Autodesk Fusion 360 part; units mm, degrees
(part 2 of 3)
  point P42 (0.5082, -2.6613)
  point P43 (0.8246, -2.9842)
  point P44 (1.3977, -3.4768)
  point P45 (1.9615, -3.8935)
  point P46 (4.9792, -5.5211)
  point P47 (9.2288, -7.083)
  point P48 (14.7308, -8.5341)
  point P49 (21.5325, -9.8694)
  point P50 (29.688, -11.1157)
  point P51 (39.2683, -12.4107)
  point P52 (50.1896, -13.9731)
  point P53 (62.2459, -15.9385)
  point P54 (75.2086, -18.3956)
  point P55 (88.7376, -21.406)
  point P56 (102.4623, -24.7749)
  point P57 (116.1281, -28.2634)
  point P58 (129.5519, -31.7626)
  point P59 (142.5417, -35.2316)
  point P60 (154.8635, -38.6462)
  point P61 (166.2937, -41.9413)
  point P62 (176.6711, -45.0342)
  point P63 (185.8834, -47.8702)
  point P64 (193.8319, -50.4036)
  point P65 (200.448, -52.5873)
  point P66 (205.676, -54.3931)
  point P67 (209.4523, -55.7878)
  point P68 (211.7241, -56.7102)
  point P69 (293.9, -147.2)
  point P70 (294.0652, -146.0004)
  point P71 (294.1279, -145.0895)
  point P72 (294.0772, -144.1146)
  point P73 (293.9994, -143.1676)
  point P74 (293.9127, -142.2878)
  point P75 (293.7566, -141.3589)
  point P76 (293.5926, -140.4177)
  point P77 (293.4026, -139.4808)
  point P78 (293.2255, -138.6248)
  point P79 (293.0974, -137.8749)
  point P80 (292.9375, -137.1059)
  point P81 (292.7021, -136.2377)
  point P82 (292.4834, -135.3764)
  point P83 (292.2718, -134.5094)
  point P84 (292.0197, -133.588)
  point P85 (291.7467, -132.6417)
  point P86 (291.4876, -131.7273)
  point P87 (291.2208, -130.8227)
  point P88 (290.9286, -129.8942)
  point P89 (290.6361, -128.9678)
  point P90 (290.3438, -128.0412)
  point P91 (290.0291, -127.0895)
  point P92 (289.6941, -126.1123)
  point P93 (289.3385, -125.1082)
  point P94 (288.9614, -124.0797)
  point P95 (288.5631, -123.025)
  point P96 (288.1588, -121.9764)
  point P97 (287.7553, -120.927)
  point P98 (287.3046, -119.8315)
  point P99 (286.8381, -118.7059)
  point P100 (286.3461, -117.5584)
  point P101 (285.8275, -116.3901)
  point P102 (285.287, -115.1981)
  point P103 (284.7, -113.9592)
  point P104 (284.1126, -112.7207)
  point P105 (283.4966, -111.4635)
  point P106 (282.8531, -110.1882)
  point P107 (282.2008, -108.9218)
  point P108 (281.514, -107.6427)
  point P109 (280.8144, -106.3767)
  point P110 (280.1033, -105.1225)
  point P111 (279.3817, -103.8791)
  point P112 (278.6514, -102.6445)
  point P113 (277.9115, -101.4197)
  point P114 (277.1545, -100.2124)
  point P115 (276.3791, -99.0239)
  point P116 (275.5907, -97.8488)
  point P117 (274.7985, -96.6775)
  point P118 (273.9974, -95.5153)
  point P119 (273.1825, -94.3673)
  point P120 (272.3507, -93.2365)
  point P121 (271.5048, -92.1202)
  point P122 (270.6449, -91.018)
  point P123 (269.7704, -89.9293)
  point P124 (268.8852, -88.853)
  point P125 (267.9907, -87.7864)
  point P126 (267.0817, -86.7346)
  point P127 (266.1565, -85.6976)
  point P128 (265.2171, -84.6768)
  point P129 (264.2633, -83.6708)
  point P130 (263.2951, -82.6778)
  point P131 (262.3106, -81.7032)
  point P132 (261.3066, -80.7468)
  point P133 (260.2862, -79.8089)
  point P134 (259.248, -78.8874)
  point P135 (258.1963, -77.9799)
  point P136 (257.1267, -77.0922)
  point P137 (256.0425, -76.2178)
  point P138 (254.9438, -75.3584)
  point P139 (253.8335, -74.5123)
  point P140 (252.7072, -73.681)
  point P141 (251.5643, -72.8667)
  point P142 (250.4037, -72.0704)
  point P143 (249.2245, -71.2932)
  point P144 (248.0274, -70.5343)
  point P145 (246.812, -69.7941)
  point P146 (245.5815, -69.0694)
  point P147 (244.3299, -68.3662)
  point P148 (243.0593, -67.6824)
  point P149 (241.7646, -67.0233)
  point P150 (240.4487, -66.3841)
  point P151 (239.1158, -65.7641)
  point P152 (237.8237, -65.1966)
  point P153 (236.6088, -64.6907)
  point P154 (235.4954, -64.2713)
  point P155 (234.4319, -63.8934)
  point P156 (233.39, -63.5413)
  point P157 (232.3995, -63.231)
  point P158 (231.4612, -62.9634)
  point P159 (230.5496, -62.7129)
  point P160 (229.667, -62.4825)
  point P161 (228.8288, -62.2994)
  point P162 (227.9917, -62.1167)
  point P163 (227.1763, -61.9564)
  point P164 (226.3862, -61.82)
  point P165 (225.5929, -61.6851)
  point P166 (224.818, -61.5795)
  point P167 (224.0639, -61.5005)
  point P168 (223.3078, -61.4218)
  point P169 (222.5837, -61.3585)
  point P170 (221.9248, -61.3226)
  point P171 (221.2934, -61.3067)
  point P172 (220.635, -61.2704)
  point P173 (220.0004, -61.2578)
  point P174 (219.4199, -61.2841)
  point P175 (218.8468, -61.3011)
  point P176 (218.2642, -61.3296)
  point P177 (217.6776, -61.3621)
  point P178 (217.0805, -61.4037)
  point P179 (216.5149, -61.4628)
  point P180 (215.9731, -61.542)
  point P181 (215.4331, -61.6212)
  point P182 (214.8778, -61.716)
  point P183 (214.3167, -61.8167)
  point P184 (213.7818, -61.937)
  point P185 (213.2797, -62.0717)
  point P186 (212.7808, -62.2013)
  point P187 (212.2834, -62.3312)
  point P188 (211.821, -62.4733)
  point P189 (211.3771, -62.6427)
  point P190 (210.9196, -62.8243)
  point P191 (210.4453, -63.0248)
  point P192 (209.9732, -63.2711)
  point P193 (209.4657, -63.5038)
  point P194 (208.9678, -63.7748)
  point P195 (208.5001, -64.0628)
  point P196 (208.135, -64.3865)
  point P197 (207.804, -64.725)
  point P198 (207.2209, -65.4396)
  point P199 (207.0786, -65.885)
  point P200 (207.1364, -66.3265)
  point P201 (207.4295, -66.7517)
  point P202 (208.4871, -67.6533)
  point P203 (209.6245, -68.4716)
  point P204 (210.8213, -69.2308)
  point P205 (212.0647, -69.9424)
  point P206 (213.3475, -70.6137)
  point P207 (214.664, -71.2504)
  point P208 (215.9986, -71.8705)
  point P209 (217.293, -72.4357)
  point P210 (218.5397, -72.9553)
  point P211 (219.7625, -73.4531)
  point P212 (220.9357, -73.9057)
  point P213 (222.0823, -74.3391)
  point P214 (223.2018, -74.754)
  point P215 (224.2923, -75.1506)
  point P216 (225.3819, -75.5481)
  point P217 (226.4707, -75.9464)
  point P218 (227.5609, -76.3433)
  point P219 (228.6442, -76.7472)
  point P220 (229.7007, -77.1306)
  point P221 (230.7539, -77.519)
  point P222 (231.8102, -77.9026)
  point P223 (232.8891, -78.311)
  point P224 (233.9682, -78.7193)
  point P225 (235.0448, -79.1301)
  point P226 (236.1446, -79.5651)
  point P227 (237.2686, -80.0217)
  point P228 (238.4157, -80.5009)
  point P229 (239.564, -80.9807)
  point P230 (240.7316, -81.4869)
  point P231 (241.9192, -82.0207)
  point P232 (243.1295, -82.5776)
  point P233 (244.3858, -83.1817)
  point P234 (245.6656, -83.8098)
  point P235 (246.9365, -84.4469)
  point P236 (248.219, -85.1185)
  point P237 (249.4891, -85.8028)
  point P238 (250.7481, -86.4984)
  point P239 (251.9963, -87.2068)
  point P240 (253.2294, -87.9289)
  point P241 (254.4466, -88.6673)
  point P242 (255.6488, -89.421)
  point P243 (256.8361, -90.1899)
  point P244 (258.0149, -90.9676)
  point P245 (259.1789, -91.7603)
  point P246 (260.3297, -92.5666)
  point P247 (261.4645, -93.3892)
  point P248 (262.5843, -94.2271)
  point P249 (263.6902, -95.0793)
  point P250 (264.7817, -95.9463)
  point P251 (265.8584, -96.8284)
  point P252 (266.9206, -97.7252)
  point P253 (267.9681, -98.6371)
  point P254 (269.004, -99.5592)
  point P255 (270.028, -100.4951)
  point P256 (271.0358, -101.4476)
  point P257 (272.0225, -102.4217)
  point P258 (272.9922, -103.4114)
  point P259 (273.9469, -104.4183)
  point P260 (274.8908, -105.4344)
  point P261 (275.817, -106.4703)
  point P262 (276.7267, -107.5215)
  point P263 (277.6214, -108.5897)
  point P264 (278.4994, -109.6732)
  point P265 (279.3581, -110.7782)
  point P266 (280.1984, -111.9003)
  point P267 (281.0184, -113.0431)
  point P268 (281.8188, -114.206)
  point P269 (282.593, -115.3975)
  point P270 (283.3408, -116.6141)
  point P271 (284.064, -117.856)
  point P272 (284.7664, -119.1191)
  point P273 (285.4525, -120.3988)
  point P274 (286.1197, -121.6963)
  point P275 (286.7489, -122.988)
  point P276 (287.3437, -124.2651)
  point P277 (287.914, -125.5228)
  point P278 (288.4388, -126.731)
  point P279 (288.9202, -127.8893)
  point P280 (289.3574, -128.9986)
  point P281 (289.7736, -130.0813)
  point P282 (290.1456, -131.115)
  point P283 (290.4959, -132.1245)
  point P284 (290.8499, -133.1303)
  point P285 (291.1589, -134.0878)
  point P286 (291.4458, -135.0199)
  point P287 (291.7397, -135.9912)
  point P288 (292.1203, -137.0555)
  point P289 (292.3769, -138.022)
  point P290 (292.6583, -139.0249)
  point P291 (292.9275, -140.0111)
  point P292 (293.1214, -140.9476)
  point P293 (293.3258, -141.8612)
  point P294 (293.4311, -142.6997)
  point P295 (293.5664, -143.5093)
  point P296 (293.6299, -144.2396)
  point P297 (293.7, -145.9)
  point P298 (293.7, -147)
  dimension "d1" = 220
  dimension "d3" = 8
  dimension "d4" = 5
  dimension "d5" = 120
  constraint coincident L0.start origin
  constraint vertical L1
  constraint perpendicular L1 L2
  constraint coincident L3.end S1.start
  measures "d1" distance of L0.start L0.end
  measures "d3" distance of L0.end L1.end
  measures "d4" distance of L1.end L2.end
  measures "d5" distance of L2.end L3.end
extrude "Extrude1" add sketch "Sketch2" along normal blind 1050 makes body 1 at (152.4021, 514.5747, 37.9525) makes body 2 at (244.5277, 405.0508, 83.2511)
sketch "Sketch3" plane through (0, 0, 0) normal (0, -1, 0) x (1, 0, 0)
  spline S0 degree 5 poles (212.4767, 57.0409) (212.4811, 57.0327) (212.4467, 56.9897) (212.2662, 56.8437) (211.8427, 56.5229) (211.2763, 56.0593) (210.7601, 55.5856) (210.2741, 55.0978) (209.7539, 54.5681) (209.168, 53.9856) (208.5221, 53.358) (207.8379, 52.7014) (207.1411, 52.0335) (206.4439, 51.3646) (205.7448, 50.6977) (205.0353, 50.0315) (204.304, 49.3629) (203.5422, 48.6889) (202.7475, 48.0094) (201.9215, 47.3254) (201.068, 46.6387) (200.192, 45.951) (199.2971, 45.2633) (198.3853, 44.5755) (197.4571, 43.8867) (196.5121, 43.1956) (195.5499, 42.5009) (194.5701, 41.8014) (193.573, 41.0967) (192.5596, 40.3867) (191.531, 39.6718) (190.4885, 38.9526) (189.4335, 38.2295) (188.367, 37.503) (187.2896, 36.7733) (186.2017, 36.0406) (185.1036, 35.3049) (183.9954, 34.5662) (182.8772, 33.8244) (181.7492, 33.0797) (180.6116, 32.3321) (179.4648, 31.5818) (178.3092, 30.8291) (177.1453, 30.0741) (175.9734, 29.3171) (174.7941, 28.5585) (173.6076, 27.7983) (172.4142, 27.037) (171.214, 26.2745) (170.0073, 25.5112) (168.7943, 24.7472) (167.575, 23.9826) (166.3497, 23.2178) (165.1186, 22.4528) (163.8818, 21.6879) (162.6396, 20.9232) (161.3921, 20.1589) (160.1396, 19.3954) (158.8823, 18.6326) (157.6203, 17.8709) (156.3539, 17.1105) (155.083, 16.3515) (153.808, 15.5943) (152.5288, 14.8389) (151.2457, 14.0856) (149.9587, 13.3347) (148.668, 12.5865) (147.3737, 11.8411) (146.076, 11.0988) (144.7749, 10.3599) (143.4707, 9.6246) (142.1634, 8.8933) (140.8531, 8.1661) (139.5399, 7.4433) (138.224, 6.725) (136.9055, 6.0116) (135.5843, 5.3032) (134.2607, 4.6001) (132.9347, 3.9025) (131.6065, 3.2107) (130.276, 2.5249) (128.9436, 1.8455) (127.6091, 1.1728) (126.2728, 0.5071) (124.9347, -0.1512) (123.5949, -0.8016) (122.2533, -1.4439) (120.9099, -2.0774) (119.5648, -2.7017) (118.2177, -3.3163) (116.8686, -3.9208) (115.5175, -4.5148) (114.1642, -5.0979) (112.8087, -5.6698) (111.4509, -6.2305) (110.0908, -6.7796) (108.7284, -7.3172) (107.3638, -7.8432) (105.9969, -8.3576) (104.6278, -8.8602) (103.2565, -9.3511) (101.8833, -9.83) (100.5082, -10.297) (99.1313, -10.7518) (97.7527, -11.1943) (96.3726, -11.6242) (94.991, -12.0415) (93.6081, -12.4458) (92.2239, -12.8369) (90.8384, -13.2148) (89.4519, -13.579) (88.0643, -13.9296) (86.6758, -14.2663) (85.2866, -14.5892) (83.8968, -14.8981) (82.5067, -15.1932) (81.1165, -15.4744) (79.7264, -15.7418) (78.3367, -15.9955) (76.9475, -16.2356) (75.5591, -16.4621) (74.1716, -16.6749) (72.7851, -16.8742) (71.4, -17.0599) (70.0162, -17.232) (68.6341, -17.3906) (67.2537, -17.5358) (65.8755, -17.6677) (64.4996, -17.7863) (63.1263, -17.8919) (61.7559, -17.9845) (60.3886, -18.0643) (59.0249, -18.1313) (57.6649, -18.1857) (56.309, -18.2276) (54.9573, -18.2569) (53.6102, -18.2736) (52.2679, -18.2779) (50.9307, -18.2696) (49.5988, -18.2488) (48.2726, -18.2154) (46.9524, -18.1694) (45.6385, -18.1109) (44.3312, -18.0398) (43.0308, -17.956) (41.7378, -17.8596) (40.4523, -17.7505) (39.1749, -17.6288) (37.9058, -17.4945) (36.6455, -17.3474) (35.3941, -17.1877) (34.1522, -17.0152) (32.92, -16.8299) (31.6978, -16.6317) (30.4861, -16.4207) (29.2853, -16.1966) (28.0958, -15.9595) (26.918, -15.7094) (25.7525, -15.4461) (24.5999, -15.1696) (23.4607, -14.8798) (22.3355, -14.5768) (21.2247, -14.2603) (20.1289, -13.9304) (19.0487, -13.587) (17.9846, -13.2299) (16.9373, -12.859) (15.9075, -12.4743) (14.896, -12.0756) (13.9038, -11.6629) (12.9318, -11.236) (11.9809, -10.7949) (11.052, -10.3396) (10.1459, -9.8701) (9.2635, -9.3866) (8.4059, -8.8889) (7.5744, -8.377) (6.7708, -7.8508) (5.9972, -7.3098) (5.2557, -6.754) (4.5484, -6.1836) (3.8771, -5.599) (3.2432, -5.0012) (2.6484, -4.3911) (2.0954, -3.7688) (1.5881, -3.1334) (1.1324, -2.4835) (0.7358, -1.8248) (0.4076, -1.1735) (0.1598, -0.566) (-0.0008, -0.0444) (-0.0815, 0.36) (-0.1201, 0.6567) (-0.145, 0.8932) (-0.1463, 1.2408) (-0.1178, 1.4667) (-0.1072, 1.5898) (-0.0507, 1.8099) (-0.0051, 1.9331) (0.0982, 2.1251) (0.1853, 2.2519) (0.289, 2.4175) (0.5475, 2.7065) (0.7064, 2.8823) (0.9696, 3.1172) (1.323, 3.4157) (1.6012, 3.648) (1.8666, 3.8408) (2.3156, 4.1171) (3.0047, 4.5094) (3.8866, 4.9842) (4.8656, 5.4778) (5.8455, 5.9275) (6.7856, 6.3085) (7.6894, 6.626) (8.585, 6.902) (9.5098, 7.1644) (10.4912, 7.4339) (11.5355, 7.7165) (12.6366, 8.0096) (13.7801, 8.3045) (14.9495, 8.591) (16.1317, 8.8613) (17.3214, 9.1127) (18.5188, 9.3462) (19.7275, 9.5655) (20.9531, 9.7752) (22.2012, 9.98) (23.475, 10.1832) (24.7753, 10.3861) (26.1011, 10.5891) (27.4501, 10.7914) (28.8195, 10.9921) (30.2063, 11.1904) (31.6084, 11.3859) (33.0247, 11.5791) (34.4546, 11.7708) (35.8983, 11.9624) (37.3562, 12.1554) (38.8286, 12.3512) (40.3159, 12.5513) (41.8181, 12.7565) (43.3347, 12.9675) (44.8651, 13.1845) (46.4085, 13.4076) (47.9638, 13.6368) (49.5301, 13.8718) (51.1066, 14.1126) (52.6927, 14.3591) (54.2877, 14.6112) (55.8914, 14.8691) (57.5035, 15.1329) (59.1238, 15.4028) (60.7521, 15.679) (62.3882, 15.962) (64.032, 16.2518) (65.6829, 16.5489) (67.3406, 16.8536) (69.0047, 17.166) (70.6745, 17.4866) (72.3495, 17.8154) (74.0292, 18.1525) (75.713, 18.498) (77.4005, 18.8518) (79.091, 19.2136) (80.7843, 19.5832) (82.4799, 19.9603) (84.1774, 20.3443) (85.8766, 20.7348) (87.5771, 21.1312) (89.2787, 21.5331) (90.9811, 21.94) (92.6841, 22.3512) (94.3874, 22.7663) (96.0908, 23.1849) (97.7942, 23.6065) (99.4973, 24.0306) (101.2001, 24.457) (102.9022, 24.8853) (104.6035, 25.3152) (106.3039, 25.7464) (108.0033, 26.1788) (109.7014, 26.6122) (111.398, 27.0465) (113.0931, 27.4815) (114.7865, 27.9172) (116.478, 28.3535) (118.1675, 28.7903) (119.8547, 29.2277) (121.5396, 29.6654) (123.2219, 30.1036) (124.9015, 30.5421) (126.5782, 30.981) (128.2518, 31.4202) (129.922, 31.8597) (131.5886, 32.2996) (133.2513, 32.7398) (134.9098, 33.1805) (136.5639, 33.6215) (138.2132, 34.063) (139.8575, 34.5051) (141.4964, 34.9476) (143.1296, 35.3908) (144.7568, 35.8345) (146.3777, 36.2789) (147.9922, 36.7238) (149.5999, 37.1693) (151.2005, 37.6154) (152.7937, 38.0619) (154.3793, 38.5087) (155.9568, 38.9557) (157.5259, 39.4027) (159.0863, 39.8495) (160.6374, 40.2958) (162.179, 40.7415) (163.7106, 41.1863) (165.232, 41.63) (166.7429, 42.0726) (168.2431, 42.514) (169.7326, 42.9541) (171.2113, 43.3932) (172.6792, 43.8311) (174.136, 44.268) (175.5817, 44.7038) (177.0156, 45.1382) (178.4372, 45.5712) (179.8454, 46.0021) (181.2394, 46.4304) (182.6181, 46.8558) (183.9806, 47.2777) (185.3264, 47.6961) (186.6553, 48.1109) (187.9678, 48.5227) (189.2648, 48.9323) (190.5471, 49.3404) (191.8152, 49.7475) (193.069, 50.1538) (194.3073, 50.5586) (195.5275, 50.9603) (196.7252, 51.3563) (197.8965, 51.744) (199.0375, 52.1213) (200.1469, 52.4876) (201.2255, 52.8442) (202.2787, 53.1956) (203.3138, 53.5477) (204.3365, 53.9054) (205.3477, 54.2702) (206.3402, 54.6382) (207.2946, 54.9968) (208.1849, 55.3291) (208.9927, 55.6238) (209.7156, 55.8811) (210.3847, 56.1254) (211.0537, 56.3976) (211.7317, 56.7089) (212.2101, 56.9445) (212.4199, 57.0387) (212.4722, 57.049) (212.4767, 57.0409) knots 0 0 0 0 0 0 0.0028169 0.0056338 0.0084507 0.01126761 0.01408451 0.01690141 0.01971831 0.02253521 0.02535211 0.02816901 0.03098592 0.03380282 0.03661972 0.03943662 0.04225352 0.04507042 0.04788732 0.05070423 0.05352113 0.05633803 0.05915493 0.06197183 0.06478873 0.06760563 0.07042254 0.07323944 0.07605634 0.07887324 0.08169014 0.08450704 0.08732394 0.09014085 0.09295775 0.09577465 0.09859155 0.10140845 0.10422535 0.10704225 0.10985915 0.11267606 0.11549296 0.11830986 0.12112676 0.12394366 0.12676056 0.12957746 0.13239437 0.13521127 0.13802817 0.14084507 0.14366197 0.14647887 0.14929577 0.15211268 0.15492958 0.15774648 0.16056338 0.16338028 0.16619718 0.16901408 0.17183099 0.17464789 0.17746479 0.18028169 0.18309859 0.18591549 0.18873239 0.1915493 0.1943662 0.1971831 0.2 0.2028169 0.2056338 0.2084507 0.21126761 0.21408451 0.21690141 0.21971831 0.22253521 0.22535211 0.22816901 0.23098592 0.23380282 0.23661972 0.23943662 0.24225352 0.24507042 0.24788732 0.25070423 0.25352113 0.25633803 0.25915493 0.26197183 0.26478873 0.26760563 0.27042254 0.27323944 0.27605634 0.27887324 0.28169014 0.28450704 0.28732394 0.29014085 0.29295775 0.29577465 0.29859155 0.30140845 0.30422535 0.30704225 0.30985915 0.31267606 0.31549296 0.31830986 0.32112676 0.32394366 0.32676056 0.32957746 0.33239437 0.33521127 0.33802817 0.34084507 0.34366197 0.34647887 0.34929577 0.35211268 0.35492958 0.35774648 0.36056338 0.36338028 0.36619718 0.36901408 0.37183099 0.37464789 0.37746479 0.38028169 0.38309859 0.38591549 0.38873239 0.3915493 0.3943662 0.3971831 0.4 0.4028169 0.4056338 0.4084507 0.41126761 0.41408451 0.41690141 0.41971831 0.42253521 0.42535211 0.42816901 0.43098592 0.43380282 0.43661972 0.43943662 0.44225352 0.44507042 0.44788732 0.45070423 0.45352113 0.45633803 0.45915493 0.46197183 0.46478873 0.46760563 0.47042254 0.47323944 0.47605634 0.47887324 0.48169014 0.48450704 0.48732394 0.49014085 0.49295775 0.49577465 0.49859155 0.50140845 0.50422535 0.50704225 0.50985915 0.51267606 0.51549296 0.51830986 0.52112676 0.52394366 0.52676056 0.52957746 0.53239437 0.53521127 0.53802817 0.54084507 0.54366197 0.54647887 0.54929577 0.55211268 0.55492958 0.55774648 0.56056338 0.56338028 0.56619718 0.56901408 0.57183099 0.57464789 0.57746479 0.58028169 0.58309859 0.58591549 0.58873239 0.5915493 0.5943662 0.5971831 0.6 0.6028169 0.6056338 0.6084507 0.61126761 0.61408451 0.61690141 0.61971831 0.62253521 0.62535211 0.62816901 0.63098592 0.63380282 0.63661972 0.63943662 0.64225352 0.64507042 0.64788732 0.65070423 0.65352113 0.65633803 0.65915493 0.66197183 0.66478873 0.66760563 0.67042254 0.67323944 0.67605634 0.67887324 0.68169014 0.68450704 0.68732394 0.69014085 0.69295775 0.69577465 0.69859155 0.70140845 0.70422535 0.70704225 0.70985915 0.71267606 0.71549296 0.71830986 0.72112676 0.72394366 0.72676056 0.72957746 0.73239437 0.73521127 0.73802817 0.74084507 0.74366197 0.74647887 0.74929577 0.75211268 0.75492958 0.75774648 0.76056338 0.76338028 0.76619718 0.76901408 0.77183099 0.77464789 0.77746479 0.78028169 0.78309859 0.78591549 0.78873239 0.7915493 0.7943662 0.7971831 0.8 0.8028169 0.8056338 0.8084507 0.81126761 0.81408451 0.81690141 0.81971831 0.82253521 0.82535211 0.82816901 0.83098592 0.83380282 0.83661972 0.83943662 0.84225352 0.84507042 0.84788732 0.85070423 0.85352113 0.85633803 0.85915493 0.86197183 0.86478873 0.86760563 0.87042254 0.87323944 0.87605634 0.87887324 0.88169014 0.88450704 0.88732394 0.89014085 0.89295775 0.89577465 0.89859155 0.90140845 0.90422535 0.90704225 0.90985915 0.91267606 0.91549296 0.91830986 0.92112676 0.92394366 0.92676056 0.92957746 0.93239437 0.93521127 0.93802817 0.94084507 0.94366197 0.94647887 0.94929577 0.95211268 0.95492958 0.95774648 0.96056338 0.96338028 0.96619718 0.96901408 0.97183099 0.97464789 0.97746479 0.98028169 0.98309859 0.98591549 0.98873239 0.9915493 0.9943662 0.9971831 1 1 1 1 1 1
  line L0 (0, 0) -> (0, -44.4339)
  line L1 (200.0276, 176.1705) -> (331.6883, 173.4705)
  line L2 (295.2866, 37.5739) -> (268.6796, 37.5739)
  line L3 (243.4554, 9.3589) -> (243.4554, -35.2869)
  line L4 (190, -75) -> (58.1049, -75)
  line L5 (0, 39.1251) -> (0, 0)
  spline S1 degree 5 poles (0, -44.4339) (0.1275, -45.1979) (0.3744, -46.6977) (0.7203, -48.8635) (1.1322, -51.5826) (1.5713, -54.6984) (1.9534, -57.5289) (2.3183, -60.0731) (2.7319, -62.3327) (3.2991, -64.3134) (4.1412, -66.0256) (5.3581, -67.4844) (6.9912, -68.7091) (8.994, -69.7244) (11.2742, -70.5573) (13.7282, -71.2365) (16.2813, -71.7898) (18.9176, -72.2433) (21.6606, -72.6209) (24.5588, -72.9436) (27.6704, -73.2293) (31.0463, -73.4924) (34.72, -73.7433) (38.7132, -73.9895) (43.0372, -74.236) (47.6968, -74.4856) (51.6931, -74.6889) (54.8407, -74.8436) (57.0057, -74.9477) (58.1049, -75) knots 0 0 0 0 0 0 0.04 0.08 0.12 0.16 0.2 0.24 0.28 0.32 0.36 0.4 0.44 0.48 0.52 0.56 0.6 0.64 0.68 0.72 0.76 0.8 0.84 0.88 0.92 0.96 1 1 1 1 1 1
  spline S2 degree 5 poles (190, -75) (190.644, -74.9855) (191.9494, -74.9359) (193.9598, -74.7996) (196.7454, -74.4938) (200.3998, -73.9045) (204.2136, -73.1128) (208.1575, -72.1327) (212.1786, -70.991) (216.1938, -69.7328) (220.1041, -68.4068) (223.8076, -67.0531) (227.2141, -65.6886) (230.2576, -64.2958) (232.9147, -62.8039) (235.1988, -61.1009) (237.1435, -59.0613) (238.791, -56.5665) (240.1771, -53.5336) (241.3272, -49.9175) (242.2591, -45.6975) (242.8386, -41.8351) (243.1822, -38.6663) (243.371, -36.4334) (243.4554, -35.2869) knots 0 0 0 0 0 0 0.05 0.1 0.15 0.2 0.25 0.3 0.35 0.4 0.45 0.5 0.55 0.6 0.65 0.7 0.75 0.8 0.85 0.9 0.95 1 1 1 1 1 1
  spline S3 degree 5 poles (243.4554, -6.3925) (243.473, -5.9904) (243.5036, -5.167) (243.5353, -3.8741) (243.5491, -2.0345) (243.5235, 0.4578) (243.4693, 3.1364) (243.4161, 5.9847) (243.416, 8.9705) (243.5375, 12.0478) (243.8539, 15.1618) (244.4331, 18.2526) (245.3276, 21.2598) (246.5615, 24.1263) (248.1272, 26.8009) (249.9974, 29.239) (252.1326, 31.4032) (254.4901, 33.2643) (257.0322, 34.803) (259.7327, 36.0111) (262.5744, 36.8872) (264.953, 37.3246) (266.7941, 37.506) (268.0469, 37.5621) (268.6796, 37.5739) knots 0 0 0 0 0 0 0.05 0.1 0.15 0.2 0.25 0.3 0.35 0.4 0.45 0.5 0.55 0.6 0.65 0.7 0.75 0.8 0.85 0.9 0.95 1 1 1 1 1 1
  line L6 (332.6837, 173.4501) -> (331.6883, 173.4705)
  line L7 (315, 114.033) -> (315, 114.033)
  line L8 (314.9907, 84.7891) -> (314.9907, 45.4342)
  spline S4 degree 2 poles (361.3602, 172.6036) (386.3573, 165.8152) (361.3602, 159.8201) knots 0 0 0 3.077992 3.077992 3.077992 weights 1 1.272727 1
  spline S5 degree 5 poles (331.4676, 173.4751) (331.4933, 173.4738) (331.5312, 173.4722) (331.5466, 173.4725) (331.6431, 173.4727) (332.3968, 173.4555) (333.9976, 173.413) (336.5222, 173.3422) (339.9458, 173.2434) (344.2007, 173.1183) (349.2053, 172.9695) (353.7523, 172.8332) (357.4473, 172.7218) (360.0351, 172.6436) (361.3602, 172.6036) knots 0 0 0 0 0 0 0.1 0.2 0.3 0.4 0.5 0.6 0.7 0.8 0.9 1 1 1 1 1 1
  line L9 (328.3992, 173.6223) -> (334.536, 173.3278)
  spline S6 degree 5 poles (340.7152, 157.4378) (341.5428, 157.5165) (343.1976, 157.6789) (345.678, 157.937) (348.9826, 158.3059) (353.1102, 158.7947) (356.4108, 159.1993) (358.8857, 159.5078) (360.5354, 159.7156) (361.3602, 159.8201) knots 0 0 0 0 0 0 0.2 0.4 0.6 0.8 1 1 1 1 1 1
  line L10 (337.7686, 157.1572) -> (343.6619, 157.7183)
  spline S7 degree 5 poles (326.5418, 156.889) (327.1441, 156.9074) (328.3406, 156.9435) (330.1113, 156.9961) (332.429, 157.0649) (335.2647, 157.1585) (337.4834, 157.2507) (339.1139, 157.3365) (340.1842, 157.4026) (340.7152, 157.4378) knots 0 0 0 0 0 0 0.2 0.4 0.6 0.8 1 1 1 1 1 1
  line L11 (326.2367, 156.8797) -> (326.8469, 156.8983)
  line L12 (340.4463, 157.4199) -> (340.9842, 157.4556)
  spline S8 degree 5 poles (326.5418, 156.889) (326.2402, 156.8699) (325.6414, 156.8355) (324.7568, 156.7953) (323.6044, 156.7649) (322.2108, 156.7618) (320.8681, 156.7821) (319.5833, 156.8019) (318.3673, 156.7804) (317.2362, 156.6538) (316.2092, 156.3481) (315.3072, 155.7978) (314.5507, 154.9612) (313.957, 153.8427) (313.54, 152.4912) (313.3105, 150.9811) (313.2765, 149.3989) (313.4428, 147.8289) (313.811, 146.3369) (314.3796, 144.963) (315.1454, 143.7299) (315.9132, 142.8637) (316.575, 142.2826) (317.0543, 141.9255) (317.3035, 141.7546) knots 0 0 0 0 0 0 0.05 0.1 0.15 0.2 0.25 0.3 0.35 0.4 0.45 0.5 0.55 0.6 0.65 0.7 0.75 0.8 0.85 0.9 0.95 1 1 1 1 1 1
  spline S9 degree 5 poles (317.3035, 141.7546) (317.4563, 141.7096) (317.7812, 141.6216) (318.3263, 141.4953) (319.1691, 141.3384) (320.4143, 141.1619) (321.8429, 141.0056) (323.4366, 140.871) (325.1617, 140.7602) (326.9749, 140.6751) (328.8293, 140.6171) (330.6797, 140.5862) (332.4889, 140.5799) (334.2333, 140.5927) (335.9087, 140.6155) (337.5243, 140.6369) (339.097, 140.645) (340.6457, 140.6293) (342.1857, 140.5824) (343.7227, 140.5016) (345.2515, 140.3893) (346.7608, 140.2509) (348.2361, 140.0931) (349.6632, 139.9229) (351.0312, 139.7455) (352.3347, 139.564) (353.324, 139.4167) (354.0356, 139.3054) (354.4965, 139.2307) (354.7236, 139.1933) knots 0 0 0 0 0 0 0.04 0.08 0.12 0.16 0.2 0.24 0.28 0.32 0.36 0.4 0.44 0.48 0.52 0.56 0.6 0.64 0.68 0.72 0.76 0.8 0.84 0.88 0.92 0.96 1 1 1 1 1 1
  spline S10 degree 2 poles (354.7236, 139.1933) (370.1413, 132.5586) (351.0765, 126.648) knots 0 0 0 2.245768 2.245768 2.245768 weights 1 1.153905 1
  spline S11 degree 5 poles (351.0765, 126.648) (351.0088, 126.6237) (350.6928, 126.5121) (350.1078, 126.3196) (349.2083, 126.0605) (347.9159, 125.7577) (346.2171, 125.4579) (344.3198, 125.2157) (342.2277, 125.0325) (339.9653, 124.9077) (337.5875, 124.837) (335.1723, 124.8135) (332.8068, 124.8277) (330.5755, 124.869) (328.5473, 124.9259) (326.7628, 124.9875) (325.2228, 125.0432) (323.8709, 125.085) (322.615, 125.1027) (321.3622, 125.0785) (320.046, 124.9824) (318.6643, 124.7641) (317.29, 124.3558) (316.0319, 123.6913) (315.0057, 122.7237) (314.302, 121.4417) (313.9528, 119.8901) (313.9428, 118.1545) (314.2264, 116.3431) (314.7426, 114.57) (315.4298, 112.9384) (316.2431, 111.5204) (317.1563, 110.3573) (317.9557, 109.6468) (318.592, 109.2402) (319.0325, 109.0252) (319.2568, 108.9317) knots 0.106418 0.106418 0.106418 0.106418 0.106418 0.106418 0.114286 0.142857 0.171429 0.2 0.228571 0.257143 0.285714 0.314286 0.342857 0.371429 0.4 0.428571 0.457143 0.485714 0.514286 0.542857 0.571429 0.6 0.628571 0.657143 0.685714 0.714286 0.742857 0.771429 0.8 0.828571 0.857143 0.885714 0.914286 0.942857 0.971429 1 1 1 1 1 1
  line L13 (354.6092, 127.9159) -> (347.5438, 125.3801)
  spline S12 degree 5 poles (319.2568, 108.9317) (319.4507, 108.9365) (319.8613, 108.9447) (320.5458, 108.9522) (321.5962, 108.9522) (323.1339, 108.9409) (324.8839, 108.9253) (326.8139, 108.9361) (328.8848, 108.9809) (331.0656, 109.0041) (333.3186, 108.9298) (335.5942, 108.6745) (337.8223, 108.1726) (339.9046, 107.3967) (341.7072, 106.3788) (343.0891, 105.1888) (343.9295, 103.9146) (344.1536, 102.6428) (343.7651, 101.4361) (342.8579, 100.3212) (341.5686, 99.3055) (340.0419, 98.3879) (338.3862, 97.5736) (336.6497, 96.8808) (334.8442, 96.3297) (332.9605, 95.9338) (330.9868, 95.691) (328.9261, 95.5741) (326.813, 95.5226) (324.7027, 95.454) (322.6632, 95.2742) (320.7653, 94.8883) (319.0745, 94.2104) (317.6404, 93.1757) (316.4939, 91.7441) (315.6529, 89.8925) (315.2306, 88.0672) (315.0556, 86.5037) (315.0019, 85.375) (314.9907, 84.7891) knots 0 0 0 0 0 0 0.028571 0.057143 0.085714 0.114286 0.142857 0.171429 0.2 0.228571 0.257143 0.285714 0.314286 0.342857 0.371429 0.4 0.428571 0.457143 0.485714 0.514286 0.542857 0.571429 0.6 0.628571 0.657143 0.685714 0.714286 0.742857 0.771429 0.8 0.828571 0.857143 0.885714 0.914286 0.942857 0.971429 1 1 1 1 1 1
  line L14 (319.645, 108.9317) -> (330.3426, 108.9317)
  spline S13 degree 5 poles (288.2629, 37.5739) (289.1719, 37.5506) (290.9605, 37.5182) (293.5557, 37.5118) (296.8373, 37.5893) (300.6186, 37.841) (304.0414, 38.2654) (307.0583, 38.8855) (309.6219, 39.7242) (311.6967, 40.7985) (313.285, 42.1074) (314.1858, 43.3328) (314.6638, 44.3471) (314.8961, 45.0649) (314.9907, 45.4342) knots 0 0 0 0 0 0 0.1 0.2 0.3 0.4 0.5 0.6 0.7 0.8 0.9 1 1 1 1 1 1
  spline S14 degree 5 poles (0, 58.174) (-0.0088, 58.3987) (-0.0254, 58.8475) (-0.0472, 59.519) (-0.0698, 60.4106) (-0.0816, 61.5158) (-0.0699, 62.3881) (-0.043, 63.0321) (-0.0159, 63.4563) (0, 63.667) knots 0 0 0 0 0 0 0.2 0.4 0.6 0.8 1 1 1 1 1 1
  line L15 (-0.0405, 63.1302) -> (0.0405, 64.2038)
  spline S15 degree 5 poles (0, 39.1251) (0.0385, 40.1788) (0.1722, 42.271) (0.5424, 45.3634) (1.3844, 49.403) (3.075, 54.3526) (5.4866, 59.2422) (8.7174, 64.0929) (12.8719, 68.8871) (18.0447, 73.5749) (24.3044, 78.0833) (31.6764, 82.3237) (40.1278, 86.2004) (49.5462, 89.6181) (59.7373, 92.4914) (70.452, 94.7561) (81.4078, 96.3809) (92.3118, 97.3787) (102.8819, 97.8185) (112.8708, 97.8385) (122.0858, 97.6548) (130.4178, 97.5845) (137.8405, 98.018) (144.3746, 99.3311) (150.0611, 101.8105) (154.9314, 105.5763) (158.9772, 110.4985) (162.127, 116.1332) (164.3102, 121.9001) (165.5217, 127.2547) (165.874, 131.8386) (165.685, 135.6973) (165.4239, 139.2201) (165.5764, 142.9106) (166.509, 147.1725) (168.4267, 152.228) (170.831, 156.9985) (173.1372, 160.9997) (174.8979, 163.8551) (175.8341, 165.3299) knots 0 0 0 0 0 0 0.028571 0.057143 0.085714 0.114286 0.142857 0.171429 0.2 0.228571 0.257143 0.285714 0.314286 0.342857 0.371429 0.4 0.428571 0.457143 0.485714 0.514286 0.542857 0.571429 0.6 0.628571 0.657143 0.685714 0.714286 0.742857 0.771429 0.8 0.828571 0.857143 0.885714 0.914286 0.942857 0.971429 1 1 1 1 1 1
  line L16 (-0.9387, 13.4558) -> (0.9387, 64.7945)
  spline S16 degree 5 poles (175.8341, 165.3299) (176.4994, 166.1201) (177.9183, 167.5965) (180.3112, 169.4992) (183.9578, 171.4982) (189.0222, 173.4002) (193.322, 174.629) (196.6407, 175.44) (198.8921, 175.9346) (200.0276, 176.1705) knots 0 0 0 0 0 0 0.2 0.4 0.6 0.8 1 1 1 1 1 1
  line L17 (174.0924, 163.2611) -> (177.5758, 167.3986)
  line L18 (196.9057, 161.1063) -> (267.6757, 157.7993)
  line L19 (196.6723, 156.1118) -> (267.4423, 152.8048)
  line L20 (196.1122, 144.1248) -> (266.8821, 140.8178)
  line L21 (195.8788, 139.1303) -> (266.6488, 135.8233)
  line L22 (195.3187, 127.1434) -> (266.0886, 123.8364)
  line L23 (195.0853, 122.1488) -> (265.8552, 118.8418)
  arc A0 (196.9057, 161.1063) -> (196.6723, 156.1118) centre (196.789, 158.609) ccw
  arc A1 (267.4423, 152.8048) -> (267.6757, 157.7993) centre (267.559, 155.302) ccw
  arc A2 (266.6488, 135.8233) -> (266.8821, 140.8178) centre (266.7655, 138.3206) ccw
  arc A3 (196.1122, 144.1248) -> (195.8788, 139.1303) centre (195.9955, 141.6276) ccw
  arc A4 (195.3187, 127.1434) -> (195.0853, 122.1488) centre (195.202, 124.6461) ccw
  arc A5 (265.8552, 118.8418) -> (266.0886, 123.8364) centre (265.9719, 121.3391) ccw
  point P0 (2.4682, -60.7962)
  point P1 (5.3006, -67.2703)
  point P2 (13.3932, -71.1142)
  point P3 (26.746, -73.1374)
  point P4 (208.0961, -72.1138)
  point P5 (228.1563, -65.2275)
  point P6 (237.7372, -58.0417)
  point P7 (243.4554, 3.9941)
  point P8 (245, 20)
  point P9 (254.1391, 32.902)
  point P10 (331.6883, 173.4705)
  point P11 (319.3481, 156.7893)
  point P12 (315, 155.4004)
  point P13 (313.4059, 148.4359)
  point P14 (322, 141)
  point P15 (332.4254, 140.5846)
  point P16 (341.3156, 140.6048)
  point P17 (349, 140)
  point P18 (341.4711, 125)
  point P19 (326.4227, 125)
  point P20 (320.4852, 125)
  point P21 (315, 122.5297)
  point P22 (315, 114.033)
  point P23 (324.9938, 108.9317)
  point P24 (337.7002, 108.1298)
  point P25 (344, 103)
  point P26 (340.4549, 98.6646)
  point P27 (331.1017, 95.7349)
  point P28 (319.939, 94.5047)
  point P29 (310, 40)
  point P30 (5.8643, 59.527)
  point P31 (37.0344, 84.6641)
  point P32 (117.8085, 97.7355)
  point P33 (154.3537, 105.5095)
  point P34 (165.5704, 129.0418)
  point P35 (165.5704, 141.0386)
  dimension "d17" = 5
  dimension "d18" = 12
  dimension "d19" = 5
  dimension "d20" = 12
  dimension "d21" = 5
  constraint vertical L0
  constraint perpendicular L2 L3
  constraint coincident L1 S16.end
  constraint coincident L1.start S16
  constraint coincident L4 S2.start
  constraint coincident S2 L4.start
  constraint coincident L3 S3.start
  constraint coincident L3 P7
  constraint coincident L2 S3.end
  constraint coincident S3 L3.start
  constraint coincident S3 L2.end
  constraint coincident L1 L6.start
  constraint parallel L1 L6
  constraint perpendicular L2 L8
  constraint coincident L6 P10
  constraint coincident L1 S5.start
  constraint midpoint S5.start L9
  constraint coincident S5 P10
  constraint midpoint S6.start L10
  constraint midpoint S7.start L11
  constraint midpoint S6.start L12
  constraint coincident L7 P22
  constraint midpoint S10.end L13
  constraint coincident S11 P22
  constraint coincident L8 S12.end
  constraint coincident S12 L8.start
  constraint midpoint P23 L14
  constraint coincident L2 S13.start
  constraint coincident S13 L2.start
  constraint coincident L5 S14.end
  constraint midpoint S14.end L15
  constraint midpoint L5.start L16
  constraint midpoint S15.end L17
  constraint tangent L19 A1
  constraint tangent L21 A3
  constraint tangent L21 A2
  constraint tangent L23 A5
  constraint tangent L23 A4